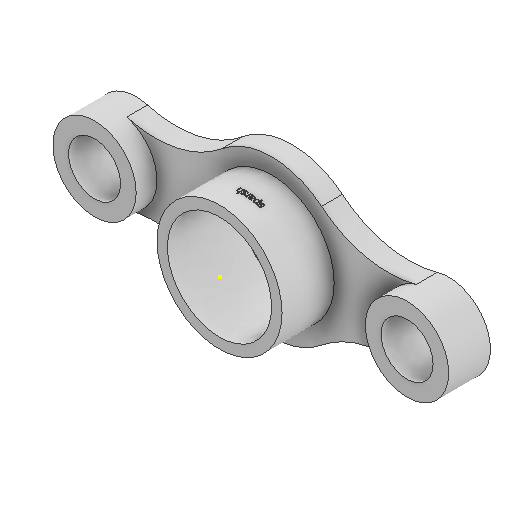
# Autodesk Inventor part: cad@72
Saved by Autodesk Inventor 2025.2 (Build 292293000, 293)
## iProperties
Created: 2025-04-22
Part Number: cad@72
Material: Generic
Document SubType Name: Modeling
Designer: spars
Density: 1 g/cm^3
Appearance: Default
Author: spars
Autodesk Inventor part; units mm, degrees
note: some values were not read from the file. Chosen so that the rebuilt part matches the saved one: direction of "Emboss1".
ref_plane "YZ Plane" through (0, 0, 0) normal (1, 0, 0) x (0, 1, 0)
sketch "Sketch1" plane through (0, 0, 0) normal (0, 0, 1) x (1, 0, 0)
  circle A0 centre (0, 0) radius 60
  circle A1 centre (0, 0) radius 50
  circle A2 centre (-150, 0) radius 25
  circle A3 centre (-150, 0) radius 40
  arc A4 (-139.0714, 38.4781) -> (-47.8929, 57.7172) centre (-111.75, 134.6734) ccw
  arc A5 (-47.8929, -57.7172) -> (-139.0714, -38.4781) centre (-111.75, -134.6734) ccw
  line L0 (0, 146.3155) -> (0, -120.9984)
  circle A6 centre (150, 0) radius 25
  circle A7 centre (150, 0) radius 40
  arc A8 (47.8929, 57.7172) -> (139.0714, 38.4781) centre (111.75, 134.6734) ccw
  arc A9 (139.0714, -38.4781) -> (47.8929, -57.7172) centre (111.75, -134.6734) ccw
  arc A10 (-47.8929, -57.7172) -> (47.8929, -57.7172) centre (0, 0) ccw
  arc A11 (47.8929, 57.7172) -> (-47.8929, 57.7172) centre (0, 0) ccw
  dimension "d0" = 120
  dimension "d1" = 100
  dimension "d3" = 50
  dimension "d4" = 80
  dimension "d6" = 150
  dimension "d8" = 200
  dimension "d9" = 100
  constraints: 16 point on circle, 12 centre point, 8 symmetric about line, 5 coincident, 2 end point, 2 tangent, 1 horizontal alignment, 1 vertical, 4 other
  measures "d0" diameter of A0
  measures "d1" diameter of A1
  measures "d3" diameter of A2
  measures "d4" diameter of A3
  measures "d6" distance of A10.centre A3.centre
  measures "d8" diameter of A4
  measures "d9" radius of A5
extrude "Extrusion1" add sketch "Sketch1" along normal blind 70 contours A0 L0 A1 | L0 A1 A0
extrude "Extrusion2" add sketch "Sketch1" along normal blind 40 contours A7 | A3
extrude "Extrusion3" add sketch "Sketch1" along normal blind 20 contours A0 L0 A11 A8 A7 A9 A10 | A0 L0 A10 A5 A3 A4 A11
sketch "Sketch2" plane through (0, 0, 70) normal (0, 0, 1) x (1, 0, 0)
  point P0 (0, 0)
ref_plane "Work Plane1" through (0, -60, 0) normal (0, 1, 0) x (-1, 0, 0)
sketch "Sketch3" plane through (0, -60, 0) normal (0, 1, 0) x (-1, 0, 0)
  line L0 (8.0663, 51.3454) -> (20.1719, 51.3454) construction
  line L1 (20.1719, 51.3454) -> (20.1719, 47.3193) construction
  line L2 (20.1719, 47.3193) -> (8.0663, 47.3193) construction
  line L3 (8.0663, 47.3193) -> (8.0663, 51.3454) construction
  point P0 (0, 0)
  constraints: 2 other
ref_plane "Work Plane2" through (0, 60, 0) normal (0, 1, 0) x (-1, 0, 0)
sketch "Sketch4" plane through (0, 60, 0) normal (0, 1, 0) x (-1, 0, 0)
  line L0 (-19.4122, 51.8364) -> (4.7989, 51.8364) construction
  line L1 (4.7989, 51.8364) -> (4.7989, 43.7841) construction
  line L2 (4.7989, 43.7841) -> (-19.4122, 43.7841) construction
  line L3 (-19.4122, 43.7841) -> (-19.4122, 51.8364) construction
  spline S0 degree 2 poles (-17.6189, 45.36) (-18.0783, 45.36) (-18.8737, 45.607) (-19.1355, 45.7453) knots 0 0 0 1 2 2 2
  line L4 (-19.1355, 45.7453) -> (-19.1355, 46.6098)
  line L5 (-19.1355, 46.6098) -> (-19.096, 46.6098)
  spline S1 degree 2 poles (-19.096, 46.6098) (-18.9972, 46.5308) (-18.7304, 46.343) (-18.5081, 46.2393) knots 0 0 0 1 2 2 2
  spline S2 degree 2 poles (-18.5081, 46.2393) (-18.3155, 46.1454) (-17.8412, 46.0071) (-17.5893, 46.0071) knots 0 0 0 1 2 2 2
  spline S3 degree 2 poles (-17.5893, 46.0071) (-17.4065, 46.0071) (-16.9866, 46.0911) (-16.8878, 46.1603) knots 0 0 0 1 2 2 2
  spline S4 degree 2 poles (-16.8878, 46.1603) (-16.7445, 46.2541) (-16.6161, 46.4665) (-16.6161, 46.6839) knots 0 0 0 1 2 2 2
  spline S5 degree 2 poles (-16.6161, 46.6839) (-16.6161, 46.9556) (-16.9125, 47.2372) (-17.2929, 47.3311) knots 0 0 0 1 2 2 2
  spline S6 degree 2 poles (-17.2929, 47.3311) (-17.4411, 47.3656) (-17.9153, 47.4644) (-18.1179, 47.5188) knots 0 0 0 1 2 2 2
  spline S7 degree 2 poles (-18.1179, 47.5188) (-18.6415, 47.6719) (-19.1158, 48.3042) (-19.1158, 48.7538) knots 0 0 0 1 2 2 2
  spline S8 degree 2 poles (-19.1158, 48.7538) (-19.1158, 49.3762) (-18.1821, 50.1518) (-17.4114, 50.1518) knots 0 0 0 1 2 2 2
  spline S9 degree 2 poles (-17.4114, 50.1518) (-17.0311, 50.1518) (-16.2604, 49.9641) (-15.9986, 49.8208) knots 0 0 0 1 2 2 2
  line L6 (-15.9986, 49.8208) -> (-15.9986, 48.9958)
  line L7 (-15.9986, 48.9958) -> (-16.0381, 48.9958)
  spline S10 degree 2 poles (-16.0381, 48.9958) (-16.3345, 49.233) (-17.0558, 49.5047) (-17.4263, 49.5047) knots 0 0 0 1 2 2 2
  spline S11 degree 2 poles (-17.4263, 49.5047) (-17.8066, 49.5047) (-18.3303, 49.1836) (-18.3303, 48.8625) knots 0 0 0 1 2 2 2
  spline S12 degree 2 poles (-18.3303, 48.8625) (-18.3303, 48.571) (-18.0191, 48.2894) (-17.6733, 48.2005) knots 0 0 0 1 2 2 2
  spline S13 degree 2 poles (-17.6733, 48.2005) (-17.5053, 48.156) (-17.0805, 48.0671) (-16.8483, 48.0128) knots 0 0 0 1 2 2 2
  spline S14 degree 2 poles (-16.8483, 48.0128) (-16.3444, 47.8843) (-15.8306, 47.2965) (-15.8306, 46.7877) knots 0 0 0 1 2 2 2
  spline S15 degree 2 poles (-15.8306, 46.7877) (-15.8306, 46.4912) (-16.0628, 45.9676) (-16.2901, 45.7749) knots 0 0 0 1 2 2 2
  spline S16 degree 2 poles (-16.2901, 45.7749) (-16.5321, 45.5724) (-17.1496, 45.36) (-17.6189, 45.36) knots 0 0 0 1 2 2 2
  spline S17 degree 2 poles (-11.2809, 47.8794) (-11.2809, 46.7333) (-12.3726, 45.3797) (-13.2075, 45.3797) knots 0 0 0 1 2 2 2
  spline S18 degree 2 poles (-13.2075, 45.3797) (-13.5483, 45.3797) (-14.072, 45.5378) (-14.3437, 45.7008) knots 0 0 0 1 2 2 2
  line L8 (-14.3437, 45.7008) -> (-14.3437, 43.7841)
  line L9 (-14.3437, 43.7841) -> (-15.1143, 43.7841)
  line L10 (-15.1143, 43.7841) -> (-15.1143, 50.0431)
  line L11 (-15.1143, 50.0431) -> (-14.3437, 50.0431)
  line L12 (-14.3437, 50.0431) -> (-14.3437, 49.5639)
  spline S19 degree 2 poles (-14.3437, 49.5639) (-14.0572, 49.8258) (-13.3557, 50.1716) (-12.9457, 50.1716) knots 0 0 0 1 2 2 2
  spline S20 degree 2 poles (-12.9457, 50.1716) (-12.1602, 50.1716) (-11.2809, 48.9267) (-11.2809, 47.8794) knots 0 0 0 1 2 2 2
  spline S21 degree 2 poles (-12.0762, 47.7905) (-12.0762, 48.5759) (-12.5752, 49.4404) (-13.1334, 49.4404) knots 0 0 0 1 2 2 2
  spline S22 degree 2 poles (-13.1334, 49.4404) (-13.4594, 49.4404) (-14.072, 49.149) (-14.3437, 48.9217) knots 0 0 0 1 2 2 2
  line L13 (-14.3437, 48.9217) -> (-14.3437, 46.3233)
  spline S23 degree 2 poles (-14.3437, 46.3233) (-14.0423, 46.18) (-13.6126, 46.0713) (-13.3359, 46.0713) knots 0 0 0 1 2 2 2
  spline S24 degree 2 poles (-13.3359, 46.0713) (-12.7382, 46.0713) (-12.0762, 46.9507) (-12.0762, 47.7905) knots 0 0 0 1 2 2 2
  spline S25 degree 2 poles (-7.9315, 45.9528) (-8.0254, 45.8836) (-8.3415, 45.6366) (-8.4897, 45.5625) knots 0 0 0 1 2 2 2
  spline S26 degree 2 poles (-8.4897, 45.5625) (-8.6923, 45.4538) (-9.0727, 45.3402) (-9.4185, 45.3402) knots 0 0 0 1 2 2 2
  spline S27 degree 2 poles (-9.4185, 45.3402) (-9.7001, 45.3402) (-10.2089, 45.5526) (-10.4015, 45.7453) knots 0 0 0 1 2 2 2
  spline S28 degree 2 poles (-10.4015, 45.7453) (-10.5843, 45.933) (-10.8066, 46.4863) (-10.8066, 46.7926) knots 0 0 0 1 2 2 2
  spline S29 degree 2 poles (-10.8066, 46.7926) (-10.8066, 47.2668) (-10.4065, 47.9387) (-9.9718, 48.1313) knots 0 0 0 1 2 2 2
  spline S30 degree 2 poles (-9.9718, 48.1313) (-9.5864, 48.3092) (-8.5391, 48.4426) (-7.9315, 48.4771) knots 0 0 0 1 2 2 2
  line L14 (-7.9315, 48.4771) -> (-7.9315, 48.6253)
  spline S31 degree 2 poles (-7.9315, 48.6253) (-7.9315, 48.8921) (-8.0945, 49.2231) (-8.2427, 49.3169) knots 0 0 0 1 2 2 2
  spline S32 degree 2 poles (-8.2427, 49.3169) (-8.3909, 49.4108) (-8.8158, 49.4701) (-9.043, 49.4701) knots 0 0 0 1 2 2 2
  spline S33 degree 2 poles (-9.043, 49.4701) (-9.3098, 49.4701) (-10.031, 49.312) (-10.3917, 49.1589) knots 0 0 0 1 2 2 2
  line L15 (-10.3917, 49.1589) -> (-10.4361, 49.1589)
  line L16 (-10.4361, 49.1589) -> (-10.4361, 49.9443)
  spline S34 degree 2 poles (-10.4361, 49.9443) (-10.2237, 50.0036) (-9.4284, 50.1518) (-9.0381, 50.1518) knots 0 0 0 1 2 2 2
  spline S35 degree 2 poles (-9.0381, 50.1518) (-8.5638, 50.1518) (-7.9167, 50.0036) (-7.6598, 49.811) knots 0 0 0 1 2 2 2
  spline S36 degree 2 poles (-7.6598, 49.811) (-7.4079, 49.6232) (-7.1609, 49.0255) (-7.1609, 48.5957) knots 0 0 0 1 2 2 2
  line L17 (-7.1609, 48.5957) -> (-7.1609, 45.4687)
  line L18 (-7.1609, 45.4687) -> (-7.9315, 45.4687)
  line L19 (-7.9315, 45.4687) -> (-7.9315, 45.9528)
  line L20 (-7.9315, 46.595) -> (-7.9315, 47.8646)
  spline S37 degree 2 poles (-7.9315, 47.8646) (-8.2082, 47.8399) (-9.043, 47.7559) (-9.3048, 47.6769) knots 0 0 0 1 2 2 2
  spline S38 degree 2 poles (-9.3048, 47.6769) (-9.6111, 47.583) (-10.0113, 47.1927) (-10.0113, 46.8469) knots 0 0 0 1 2 2 2
  spline S39 degree 2 poles (-10.0113, 46.8469) (-10.0113, 46.4517) (-9.5667, 46.0516) (-9.1418, 46.0516) knots 0 0 0 1 2 2 2
  spline S40 degree 2 poles (-9.1418, 46.0516) (-8.7812, 46.0516) (-8.1884, 46.3628) (-7.9315, 46.595) knots 0 0 0 1 2 2 2
  line L21 (-3.6535, 49.2181) -> (-3.693, 49.2181)
  spline S41 degree 2 poles (-3.693, 49.2181) (-3.7819, 49.2428) (-3.9746, 49.2527) (-4.1079, 49.2527) knots 0 0 0 1 2 2 2
  spline S42 degree 2 poles (-4.1079, 49.2527) (-4.4192, 49.2527) (-5.0317, 48.981) (-5.3084, 48.7143) knots 0 0 0 1 2 2 2
  line L22 (-5.3084, 48.7143) -> (-5.3084, 45.4687)
  line L23 (-5.3084, 45.4687) -> (-6.079, 45.4687)
  line L24 (-6.079, 45.4687) -> (-6.079, 50.0431)
  line L25 (-6.079, 50.0431) -> (-5.3084, 50.0431)
  line L26 (-5.3084, 50.0431) -> (-5.3084, 49.3614)
  spline S43 degree 2 poles (-5.3084, 49.3614) (-4.8885, 49.7369) (-4.2611, 50.0431) (-3.9647, 50.0431) knots 0 0 0 1 2 2 2
  spline S44 degree 2 poles (-3.9647, 50.0431) (-3.8461, 50.0431) (-3.7276, 50.0333) (-3.6535, 50.0184) knots 0 0 0 1 2 2 2
  line L27 (-3.6535, 50.0184) -> (-3.6535, 49.2181)
  spline S45 degree 2 poles (-1.8207, 45.36) (-2.2801, 45.36) (-3.0755, 45.607) (-3.3373, 45.7453) knots 0 0 0 1 2 2 2
  line L28 (-3.3373, 45.7453) -> (-3.3373, 46.6098)
  line L29 (-3.3373, 46.6098) -> (-3.2978, 46.6098)
  spline S46 degree 2 poles (-3.2978, 46.6098) (-3.199, 46.5308) (-2.9322, 46.343) (-2.7099, 46.2393) knots 0 0 0 1 2 2 2
  spline S47 degree 2 poles (-2.7099, 46.2393) (-2.5172, 46.1454) (-2.043, 46.0071) (-1.7911, 46.0071) knots 0 0 0 1 2 2 2
  spline S48 degree 2 poles (-1.7911, 46.0071) (-1.6083, 46.0071) (-1.1884, 46.0911) (-1.0896, 46.1603) knots 0 0 0 1 2 2 2
  spline S49 degree 2 poles (-1.0896, 46.1603) (-0.9463, 46.2541) (-0.8179, 46.4665) (-0.8179, 46.6839) knots 0 0 0 1 2 2 2
  spline S50 degree 2 poles (-0.8179, 46.6839) (-0.8179, 46.9556) (-1.1143, 47.2372) (-1.4947, 47.3311) knots 0 0 0 1 2 2 2
  spline S51 degree 2 poles (-1.4947, 47.3311) (-1.6429, 47.3656) (-2.1171, 47.4644) (-2.3196, 47.5188) knots 0 0 0 1 2 2 2
  spline S52 degree 2 poles (-2.3196, 47.5188) (-2.8433, 47.6719) (-3.3175, 48.3042) (-3.3175, 48.7538) knots 0 0 0 1 2 2 2
  spline S53 degree 2 poles (-3.3175, 48.7538) (-3.3175, 49.3762) (-2.3839, 50.1518) (-1.6132, 50.1518) knots 0 0 0 1 2 2 2
  spline S54 degree 2 poles (-1.6132, 50.1518) (-1.2328, 50.1518) (-0.4622, 49.9641) (-0.2004, 49.8208) knots 0 0 0 1 2 2 2
  line L30 (-0.2004, 49.8208) -> (-0.2004, 48.9958)
  line L31 (-0.2004, 48.9958) -> (-0.2399, 48.9958)
  spline S55 degree 2 poles (-0.2399, 48.9958) (-0.5363, 49.233) (-1.2575, 49.5047) (-1.628, 49.5047) knots 0 0 0 1 2 2 2
  spline S56 degree 2 poles (-1.628, 49.5047) (-2.0084, 49.5047) (-2.5321, 49.1836) (-2.5321, 48.8625) knots 0 0 0 1 2 2 2
  spline S57 degree 2 poles (-2.5321, 48.8625) (-2.5321, 48.571) (-2.2208, 48.2894) (-1.875, 48.2005) knots 0 0 0 1 2 2 2
  spline S58 degree 2 poles (-1.875, 48.2005) (-1.7071, 48.156) (-1.2822, 48.0671) (-1.0501, 48.0128) knots 0 0 0 1 2 2 2
  spline S59 degree 2 poles (-1.0501, 48.0128) (-0.5462, 47.8843) (-0.0324, 47.2965) (-0.0324, 46.7877) knots 0 0 0 1 2 2 2
  spline S60 degree 2 poles (-0.0324, 46.7877) (-0.0324, 46.4912) (-0.2646, 45.9676) (-0.4918, 45.7749) knots 0 0 0 1 2 2 2
  spline S61 degree 2 poles (-0.4918, 45.7749) (-0.7339, 45.5724) (-1.3514, 45.36) (-1.8207, 45.36) knots 0 0 0 1 2 2 2
  line L32 (4.2753, 45.4687) -> (3.5047, 45.4687)
  line L33 (3.5047, 45.4687) -> (3.5047, 48.077)
  spline S62 degree 2 poles (3.5047, 48.077) (3.5047, 48.3932) (3.4454, 48.9366) (3.3565, 49.0996) knots 0 0 0 1 2 2 2
  spline S63 degree 2 poles (3.3565, 49.0996) (3.2626, 49.2725) (2.9267, 49.4404) (2.6401, 49.4404) knots 0 0 0 1 2 2 2
  spline S64 degree 2 poles (2.6401, 49.4404) (2.3536, 49.4404) (1.746, 49.1342) (1.4545, 48.8872) knots 0 0 0 1 2 2 2
  line L34 (1.4545, 48.8872) -> (1.4545, 45.4687)
  line L35 (1.4545, 45.4687) -> (0.6839, 45.4687)
  line L36 (0.6839, 45.4687) -> (0.6839, 51.8364)
  line L37 (0.6839, 51.8364) -> (1.4545, 51.8364)
  line L38 (1.4545, 51.8364) -> (1.4545, 49.5343)
  spline S65 degree 2 poles (1.4545, 49.5343) (1.8003, 49.8455) (2.4672, 50.1716) (2.8427, 50.1716) knots 0 0 0 1 2 2 2
  spline S66 degree 2 poles (2.8427, 50.1716) (3.5145, 50.1716) (4.2753, 49.2824) (4.2753, 48.4376) knots 0 0 0 1 2 2 2
  line L39 (4.2753, 48.4376) -> (4.2753, 45.4687)
  point P0 (0, 0)
  constraints: 2 other
emboss "Emboss1" sketch "Sketch4" operation cut depth 10 direction (0, -1, 0)
body "Solid1"
